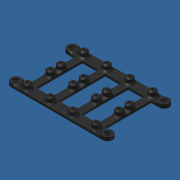
# Autodesk Inventor part: MotorDriverMount
Saved by Autodesk Inventor 2014 SP2 (Build 180246200, 246)
## iProperties
Created: 2015-02-22
Part Number: MotorDriverMount
Material: ABS-Kunststoff - Schwarz
Document SubType Name: Modeling
Designer: 4ndreas
Density: 1.06 g/cm^3
Appearance: Glatt - weiß(2)
Author: 4ndreas
Autodesk Inventor part; units mm, degrees
ref_plane "YZ Plane" through (0, 0, 0) normal (1, 0, 0) x (0, 1, 0)
ref_plane "XZ Plane" through (0, 0, 0) normal (0, 1, 0) x (-1, 0, 0)
sketch "Skizze1" plane through (0, 0, 0) normal (0, 0, 1) x (1, 0, 0)
  circle A0 centre (-65, -39.9989) radius 2 projected
  circle A1 centre (65, 40.0011) radius 2 projected
  circle A2 centre (65, -39.9989) radius 2 projected
  circle A3 centre (-65, 40.0011) radius 2 projected
  line L0 (-80, -49.9989) -> (-72, -49.9989) projected
  line L1 (-72, -49.9989) -> (-72, -60.3935) projected
  line L2 (-72, -60.3935) -> (72, -60.3935) projected
  line L3 (72, -60.3935) -> (72, -49.9989) projected
  line L4 (72, -49.9989) -> (80, -49.9989) projected
  line L5 (80, -49.9989) -> (80, 50.0011) projected
  line L6 (80, 50.0011) -> (72, 50.0011) projected
  line L7 (72, 50.0011) -> (72, 60.3935) projected
  line L8 (72, 60.3935) -> (-72, 60.3935) projected
  line L9 (-72, 60.3935) -> (-72, 50.0011) projected
  line L10 (-72, 50.0011) -> (-80, 50.0011) projected
  line L11 (-80, 50.0011) -> (-80, -49.9989) projected
  line L12 (-65, -39.9989) -> (65, -39.9989) construction
  line L13 (-65, -46.9989) -> (65, -46.9989)
  line L14 (65, -32.9989) -> (-65, -32.9989)
  arc A4 (-65, -32.9989) -> (-65, -46.9989) centre (-65, -39.9989) ccw
  arc A5 (65, -46.9989) -> (65, -32.9989) centre (65, -39.9989) ccw
  line L15 (65, 40.0011) -> (-65, 40.0011) construction
  line L16 (65, 47.0011) -> (-65, 47.0011)
  line L17 (-65, 33.0011) -> (65, 33.0011)
  arc A6 (65, 33.0011) -> (65, 47.0011) centre (65, 40.0011) ccw
  arc A7 (-65, 47.0011) -> (-65, 33.0011) centre (-65, 40.0011) ccw
  line L18 (-53.75, -32.9989) -> (-43.75, -32.9989)
  line L19 (-43.75, -32.9989) -> (-43.75, 33.0011)
  line L20 (-43.75, 33.0011) -> (-53.75, 33.0011)
  line L21 (-53.75, 33.0011) -> (-53.75, -32.9989)
  line L22 (-21.25, -32.9989) -> (-11.25, -32.9989)
  line L23 (-11.25, -32.9989) -> (-11.25, 33.0011)
  line L24 (-11.25, 33.0011) -> (-21.25, 33.0011)
  line L25 (-21.25, 33.0011) -> (-21.25, -32.9989)
  line L26 (59.2651, -32.9989) -> (51.7998, -32.9989)
  line L27 (51.7998, 33.0011) -> (59.2651, 33.0011)
  line L28 (33.6966, -32.9989) -> (24.8316, -32.9989)
  line L29 (24.8316, 33.0011) -> (33.6966, 33.0011)
  line L30 (0, -39.9989) -> (0, 40.0011) construction
  line L31 (-32.5, -39.9989) -> (-32.5, 40.0011) construction
  line L32 (-65, -39.9989) -> (-65, 40.0011) construction
  line L33 (-48.75, -39.9989) -> (-48.75, 40.0011) construction
  line L34 (-16.25, -39.9989) -> (-16.25, 40.0011) construction
  point P0 (0, 0)
  dimension "d0" = 32.5
  dimension "d1" = 10
  constraints: 50 end point, 14 point on line, 12 parallel, 10 tangent, 8 point on circle, 4 centre point, 4 horizontal, 4 perpendicular, 2 midpoint, 5 other
  measures "d0" distance between parallel lines of L34 L33
  measures "d1" distance between parallel lines of L19 L21
extrude "Extrusion1" add sketch "Skizze1" along normal blind 3 contours A4 L14 A5 L13 | L21 L17 L19 L14 | L17 A7 L16 A6 | L25 L17 L23 L14
sketch "Skizze2" plane through (0, 0, 3) normal (0, 0, 1) x (1, 0, 0)
  line L0 (-43.75, -32.9989) -> (-43.75, 33.0011) projected
  line L1 (-11.25, -32.9989) -> (-11.25, 33.0011) projected
  line L2 (-48.75, -39.9989) -> (-48.75, 40.0011) construction
  line L3 (-16.25, -39.9989) -> (-16.25, 40.0011) construction
  line L4 (-65, -39.9989) -> (65, -39.9989) construction
  line L5 (65, 40.0011) -> (-65, 40.0011) construction
  circle A0 centre (-48.75, -39.9989) radius 5
  circle A1 centre (-16.25, -39.9989) radius 5
  circle A2 centre (-16.25, 40.0011) radius 5
  circle A3 centre (-48.75, 40.0011) radius 5
  circle A4 centre (-48.75, -7.4989) radius 5
  circle A5 centre (-48.75, 7.5011) radius 5
  circle A6 centre (-16.25, -7.4989) radius 5
  circle A7 centre (-16.25, 7.5011) radius 5
  line L6 (-16.25, -7.4989) -> (-48.75, -7.4989) construction
  line L7 (-16.25, 7.5011) -> (-48.75, 7.5011) construction
  point P0 (0, 0)
  dimension "d4" = 32.5
  dimension "d5" = 32.5
  constraints: 8 centre point, 5 coincident, 4 end point, 4 equal radius, 4 point on line, 4 tangent, 2 perpendicular
  measures "d4" distance between parallel lines of L4 L6
  measures "d5" distance between parallel lines of L7 L5
extrude "Extrusion2" add sketch "Skizze2" along normal blind 8
chamfer "Fase1" distance 1.5 angle 45 8 edges at (-21.25, -39.9989, 11) (-53.75, -39.9989, 11) (-53.75, -7.4989, 11) (-21.25, -7.4989, 11) (-21.25, 7.5011, 11) (-21.25, 40.0011, 11) (-53.75, 40.0011, 11) (-53.75, 7.5011, 11)
sketch "Skizze4" plane through (0, 0, 0) normal (0, 0, -1) x (-1, 0, 0)
  line L0 (53.75, -32.9989) -> (65, -32.9989) projected
  circle A0 centre (16.25, -39.9989) radius 5 projected
  circle A1 centre (16.25, -39.9989) radius 3.5 projected
  circle A2 centre (16.25, -7.4989) radius 3.5 projected
  circle A3 centre (16.25, 7.5011) radius 3.5 projected
  circle A4 centre (16.25, 40.0011) radius 3.5 projected
  circle A5 centre (48.75, 40.0011) radius 3.5 projected
  circle A6 centre (48.75, 7.5011) radius 3.5 projected
  circle A7 centre (48.75, -7.4989) radius 3.5 projected
  circle A8 centre (48.75, -39.9989) radius 3.5 projected
  point P0 (0, 0)
hole "Bohrung1" at (-48.75, 40.0011, 0) at (-16.25, 40.0011, 0) at (-16.25, 7.5011, 0) at (-48.75, 7.5011, 0) at (-48.75, -7.4989, 0) at (-16.25, -7.4989, 0) at (-16.25, -39.9989, 0) at (-48.75, -39.9989, 0) direction (0, 0, 1) diameter 3 end through all counterbore diameter 6 counterbore depth 2
sketch "Skizze5" plane through (-48.75, 40.0011, 2) normal (0, 0, -1) x (-1, 0, 0)
  circle A0 centre (0, 0) radius 1.5
  circle A1 centre (-32.5, 0) radius 3
  circle A2 centre (-32.5, 0) radius 1.5
  circle A3 centre (-32.5, -32.5) radius 3
  circle A4 centre (-32.5, -32.5) radius 1.5
  circle A5 centre (-32.5, -47.5) radius 3
  circle A6 centre (-32.5, -47.5) radius 1.5
  circle A7 centre (0, -47.5) radius 3
  circle A8 centre (0, -47.5) radius 1.5
  circle A9 centre (0, -80) radius 3
  circle A10 centre (0, -80) radius 1.5
  circle A11 centre (-32.5, -80) radius 3
  circle A12 centre (-32.5, -80) radius 1.5
  circle A13 centre (0, -32.5) radius 1.5
  circle A14 centre (0, -32.5) radius 1.5
  point P0 (-48.75, -40.0011)
extrude "Extrusion3" add sketch "Skizze5" against normal blind 0.4 contours A0 | A2 | A4 | A6 | A8 | A10 | A12 | A13
sketch "Skizze6" plane through (0, 0, 3) normal (0, 0, 1) x (1, 0, 0)
  line L0 (-53.75, -32.9989) -> (-65, -32.9989) projected
  arc A0 (-65, -32.9989) -> (-65, -46.9989) centre (-65, -39.9989) ccw projected
  circle A1 centre (-65, -39.9989) radius 2 projected
  circle A2 centre (-16.25, 40.0011) radius 5 projected
  circle A3 centre (-48.75, 40.0011) radius 5 projected
  circle A4 centre (-65, 40.0011) radius 2 projected
  circle A5 centre (65, 40.0011) radius 2 projected
  arc A6 (-43.75, 7.5011) -> (-53.75, 7.5011) centre (-48.75, 7.5011) ccw projected
  line L1 (-43.75, 7.5011) -> (-43.75, 33.0011) projected
  line L2 (-43.75, 33.0011) -> (-21.25, 33.0011) projected
  line L3 (-21.25, 33.0011) -> (-21.25, 7.5011) projected
  arc A7 (-11.25, 7.5011) -> (-21.25, 7.5011) centre (-16.25, 7.5011) ccw projected
  line L4 (-11.25, 7.5011) -> (-11.25, 33.0011) projected
  line L5 (-11.25, 33.0011) -> (65, 33.0011) projected
  arc A8 (65, 33.0011) -> (65, 47.0011) centre (65, 40.0011) ccw projected
  line L6 (65, 47.0011) -> (-65, 47.0011) projected
  arc A9 (-65, 47.0011) -> (-65, 33.0011) centre (-65, 40.0011) ccw projected
  line L7 (-65, 33.0011) -> (-53.75, 33.0011) projected
  line L8 (-53.75, 33.0011) -> (-53.75, 7.5011) projected
  line L9 (-67.0207, -36.4989) -> (-62.9793, -36.4989)
  line L10 (-62.9793, -36.4989) -> (-60.9585, -39.9989)
  line L11 (-60.9585, -39.9989) -> (-62.9793, -43.4989)
  line L12 (-62.9793, -43.4989) -> (-67.0207, -43.4989)
  line L13 (-67.0207, -43.4989) -> (-69.0415, -39.9989)
  line L14 (-69.0415, -39.9989) -> (-67.0207, -36.4989)
  line L15 (-67.0207, 36.5011) -> (-69.0415, 40.0011)
  line L16 (-69.0415, 40.0011) -> (-67.0207, 43.5011)
  line L17 (-67.0207, 43.5011) -> (-62.9793, 43.5011)
  line L18 (-62.9793, 43.5011) -> (-60.9585, 40.0011)
  line L19 (-60.9585, 40.0011) -> (-62.9793, 36.5011)
  line L20 (-62.9793, 36.5011) -> (-67.0207, 36.5011)
  circle A10 centre (-65, 40.0011) radius 7
  circle A11 centre (-65, -39.9989) radius 7
  point P0 (0, 0)
  dimension "d20" = 7
  constraints: 24 end point, 4 coincident, 3 parallel, 2 centre point, 2 concentric, 26 other
  measures "d20" distance between parallel lines of L20 L17
extrude "Extrusion4" add sketch "Skizze6" along normal blind 2 contours A11 A0 | A9 A10
chamfer "Fase2" distance 2 angle 45 4 edges at (-60.0503, -44.9486, 3) (-60.0503, -35.0491, 3) (-60.0503, 35.0514, 3) (-60.0503, 44.9509, 3)
ref_plane "Arbeitsebene1" through (0, -39.9989, 0) normal (1, 0, 0) x (0, 1, 0)
chamfer "Fase3" distance 2 angle 45 12 edges at (-53.75, -39.9989, 3) (-21.25, -39.9989, 3) (-16.25, -12.4989, 3) (-48.75, -12.4989, 3) (-48.75, -2.4989, 3) (-16.25, -2.4989, 3) (-16.25, 2.5011, 3) (-16.25, 12.5011, 3) (-48.75, 12.5011, 3) (-48.75, 2.5011, 3) (-21.25, 40.0011, 3) (-53.75, 40.0011, 3)
split "Trennen1" plane through (0, -39.9989, 0) removes the side toward (1, 0, 0)
mirror "Spiegeln1" about plane through (0, 0, 0) normal (1, 0, 0)
equation "\"d4\" = d0"
equation "\"d5\" = d4"
